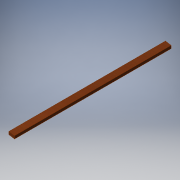
# Autodesk Inventor part: Back 2x4
Saved by Autodesk Inventor 2016 (Build 200138000, 138)
## iProperties
Created: 2015-07-07
Part Number: Back 2x4
Material: Wood (Walnut)
Document SubType Name: Modeling
Designer: steele
Density: 0.55 g/cm^3
Appearance: Walnut - Natural Polished
Author: steele
Autodesk Inventor part; units mm, degrees
ref_plane "YZ Plane" through (0, 0, 0) normal (1, 0, 0) x (0, 1, 0)
ref_plane "XZ Plane" through (0, 0, 0) normal (0, 1, 0) x (-1, 0, 0)
ref_plane "XY Plane" through (0, 0, 0) normal (0, 0, 1) x (1, 0, 0)
sketch "Sketch1" plane through (0, 0, 0) normal (0, 1, 0) x (-1, 0, 0)
  line L0 (-44.45, 1047.242) -> (-44.45, -1047.242)
  line L1 (-44.45, -1047.242) -> (44.45, -1047.242)
  line L2 (44.45, -1047.242) -> (44.45, 1047.242)
  line L3 (44.45, 1047.242) -> (-44.45, 1047.242)
  line L4 (-44.45, 1047.242) -> (44.45, -1047.242) construction
  line L5 (-44.45, -1047.242) -> (44.45, 1047.242) construction
  point P0 (0, 0)
  dimension "d0" = 2094.484
  dimension "d1" = 88.9
  constraints: 12 end point, 2 midpoint, 2 parallel, 1 perpendicular, 1 vertical
  measures "d0" distance of L1.end L2.end
  measures "d1" distance of L2.end L0.start
extrude "Extrusion1" add sketch "Sketch1" along normal blind 38.1
sketch "Sketch4" plane through (0, 38.1, 0) normal (0, 1, 0) x (1, 0, 0)
  line L0 (-44.45, 1047.242) -> (-44.45, -1047.242) projected
  line L1 (-44.45, -1047.242) -> (44.45, -1061.3224)
  line L2 (44.45, -1047.242) -> (44.45, 1047.242) projected
  line L3 (44.45, -1061.3224) -> (44.45, -1047.242)
  line L4 (-44.45, -1047.242) -> (44.45, -1047.242) projected
  point P0 (0, 0)
  dimension "d8" = 9
  constraints: 4 end point, 1 collinear
  measures "d8" angle of L1 L4
extrude "Extrusion3" add sketch "Sketch4" against normal blind 38.1
sketch "Sketch5" plane through (0, 38.1, 0) normal (0, 1, 0) x (1, 0, 0)
  line L0 (44.45, -1061.3224) -> (44.45, 1047.242) projected
  line L1 (44.45, 1047.242) -> (-44.45, 1061.3224)
  line L2 (44.45, 1047.242) -> (-44.45, 1047.242) projected
  line L3 (-44.45, 1061.3224) -> (-44.45, 1047.242)
  line L4 (-44.45, 1047.242) -> (44.45, 1047.242)
  line L5 (-44.45, 1047.242) -> (-44.45, -1047.242) projected
  point P0 (0, 0)
  dimension "d11" = 9
  constraints: 6 end point, 2 collinear
  measures "d11" angle of L1 L2
extrude "Extrusion4" add sketch "Sketch5" against normal blind 38.1
body "Solid1"
